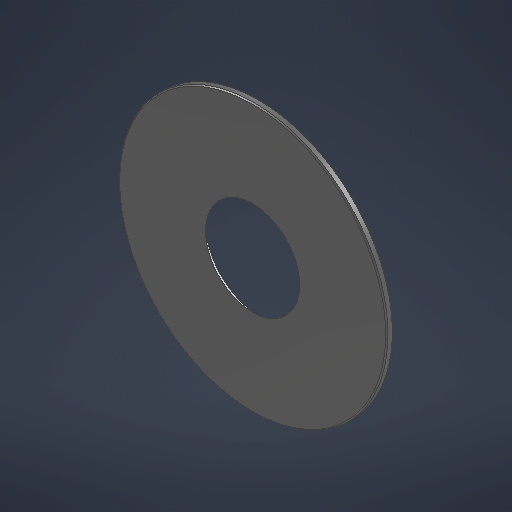
# Autodesk Inventor part: spool_side
Saved by Autodesk Inventor 2026.1 (Build 301233000, 233)
## iProperties
Created: 2023-11-23
Part Number: spool_side
Material: Generic
Document SubType Name: Modeling
Designer: aaron
Density: 1 g/cm^3
Appearance: Default
Author: aaron
Autodesk Inventor part; units mm, degrees
ref_plane "YZ Plane" through (0, 0, 0) normal (1, 0, 0) x (0, 1, 0)
ref_plane "XZ Plane" through (0, 0, 0) normal (0, 1, 0) x (-1, 0, 0)
ref_plane "XY Plane" through (0, 0, 0) normal (0, 0, 1) x (1, 0, 0)
sketch "Sketch1" plane through (0, 0, 0) normal (0, 0, 1) x (1, 0, 0)
  circle A0 centre (0, 0) radius 60
  dimension "d0" = 120
  constraints: 1 centre point, 1 coincident
  measures "d0" diameter of A0
extrude "Extrusion1" add sketch "Sketch1" along normal blind 3
chamfer "Chamfer2" distance 0.5 angle 45 2 edges at (-60, 0, 3) (-60, 0, 0)
sketch "Sketch5" plane through (0, 0, 3) normal (0, 0, 1) x (1, 0, 0)
  circle A0 centre (0, 0) radius 21.05
  dimension "d36" = 42.1
  constraints: 1 centre point, 1 coincident
  measures "d36" diameter of A0
extrude "Extrusion5" cut sketch "Sketch5" against normal through all
chamfer "Chamfer3" distance 3 angle 45 1 edges at (-21.05, 0, 0)
body "Solid1"
